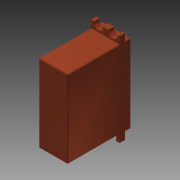
# Autodesk Inventor part: Serwo
Saved by Autodesk Inventor 2014 (Build 180170000, 170)
## iProperties
Created: 2013-10-14
Part Number: Serwo
Material: Miedź
Document SubType Name: Modeling
Designer: Wojciech
Density: 8.94 g/cm^3
Appearance: Miedź - satynowa
Author: Wojciech
Autodesk Inventor part; units mm, degrees
ref_plane "YZ Plane" through (0, 0, 0) normal (1, 0, 0) x (0, 1, 0)
ref_plane "XZ Plane" through (0, 0, 0) normal (0, 1, 0) x (-1, 0, 0)
ref_plane "XY Plane" through (0, 0, 0) normal (0, 0, 1) x (1, 0, 0)
sketch "Szkic1" plane through (0, 0, 0) normal (0, 1, 0) x (-1, 0, 0)
  line L0 (-10, 27) -> (10, 27)
  line L1 (10, 27) -> (10, -27)
  line L2 (10, -27) -> (-10, -27)
  line L3 (-10, -27) -> (-10, 27)
  line L4 (-10, 27) -> (10, -27) construction
  line L5 (10, 27) -> (-10, -27) construction
  point P0 (0, 0)
  dimension "d0" = 20
  dimension "d1" = 54
  constraints: 12 end point, 2 midpoint, 2 parallel, 1 horizontal, 1 perpendicular
  measures "d0" distance of L1.end L2.end
  measures "d1" distance of L0.end L1.end
extrude "Wyciągnięcie proste1" add sketch "Szkic1" along normal blind 36
sketch "Szkic2" plane through (0, 36, 0) normal (0, 1, 0) x (1, 0, 0)
  line L0 (-10, -27) -> (10, -27) projected
  line L1 (10, -27) -> (10, 27) projected
  line L2 (10, 27) -> (-10, 27) projected
  line L3 (-10, 27) -> (-10, -27) projected
  line L4 (-10, -27) -> (-10, -32)
  line L5 (-10, -32) -> (10, -32)
  line L6 (10, -32) -> (10, -27)
  line L7 (10, 27) -> (10, 32)
  line L8 (10, 32) -> (-10, 32)
  line L9 (-10, 32) -> (-10, 27)
  circle A0 centre (-5.0245, -32) radius 3
  circle A1 centre (5.0062, -32) radius 3
  circle A2 centre (-5.0245, 32) radius 3
  circle A3 centre (5.0062, 32) radius 3
  point P0 (0, 0)
  dimension "d4" = 5
  dimension "d5" = 5
  dimension "d8" = 6
  dimension "d9" = 6
  dimension "d10" = 6
  dimension "d11" = 6
  constraints: 12 end point, 4 centre point, 4 point on line, 3 perpendicular, 2 collinear, 1 coincident, 1 parallel
  measures "d4" distance of L0.start L4.end
  measures "d5" distance of L1.end L7.end
  measures "d8" diameter of A0
  measures "d9" diameter of A1
  measures "d10" diameter of A2
  measures "d11" diameter of A3
extrude "Wyciągnięcie proste2" add sketch "Szkic2" along normal blind 4 contours L3 L2 L1 L0 | L0 L6 L5 A1 A0 L4 | L9 L8 A2 A3 L7 L2 | A0 L5 | L5 A1 | L8 A2 | A3 L8 picked at (-4.1905, -30.6328) picked at (5.8402, -30.6328) picked at (-5.5926, 30.2476) picked at (4.4381, 30.2476)
hole "Otwór1" at (5.2587, 40, 31.3846) direction (0, -1, 0) diameter 6 depth 8 tip angle 118
hole "Otwór2" at (-4.8112, 40, 31.2727) direction (0, -1, 0) diameter 6 depth 8 tip angle 118
hole "Otwór3" at (4.5874, 40, -30.3776) direction (0, -1, 0) diameter 6 depth 8 tip angle 118
hole "Otwór4" at (-4.6993, 40, -30.4895) direction (0, -1, 0) diameter 6 depth 8 tip angle 118
sketch "Szkic3" plane through (0, 40, 0) normal (0, 1, 0) x (1, 0, 0)
  line L0 (-10, 27) -> (10, 27)
  line L1 (10, 27) -> (10, -27)
  line L2 (10, -27) -> (-10, -27)
  line L3 (-10, -27) -> (-10, 27)
  line L4 (-10, 27) -> (10, -27) construction
  line L5 (10, 27) -> (-10, -27) construction
  point P0 (0, 0)
  dimension "d48" = 20
  dimension "d49" = 54
  constraints: 12 end point, 2 midpoint, 2 parallel, 1 horizontal, 1 perpendicular
  measures "d48" distance of L1.end L2.end
  measures "d49" distance of L0.end L1.end
extrude "Wyciągnięcie proste3" add sketch "Szkic3" along normal blind 4
sketch "Szkic4" plane through (0, 44, 0) normal (0, 1, 0) x (1, 0, 0)
  line L0 (-8.5229, 17.6007) -> (8.5229, 17.6007)
  line L1 (8.5229, 17.6007) -> (8.5229, 0)
  line L2 (8.5229, 0) -> (-8.5229, 0)
  line L3 (-8.5229, 0) -> (-8.5229, 17.6007)
  line L4 (-8.5229, 17.6007) -> (8.5229, 0) construction
  line L5 (8.5229, 17.6007) -> (-8.5229, 0) construction
  arc A0 (8.5229, 17.6007) -> (-8.5229, 17.6007) centre (0, 17.6007) ccw
  point P0 (0, 0)
  point P1 (0, 8.8003)
  constraints: 12 end point, 2 midpoint, 2 parallel, 2 point on circle, 2 tangent, 1 centre point, 1 horizontal, 1 perpendicular
extrude "Wyciągnięcie proste4" add sketch "Szkic4" along normal blind 1
sketch "Szkic5" plane through (0, 45, 0) normal (0, 1, 0) x (1, 0, 0)
  arc A0 (8.5229, 17.6007) -> (-8.5229, 17.6007) centre (0, 17.6007) ccw projected
  circle A1 centre (0, 17.6007) radius 5
  point P0 (0, 0)
  dimension "d54" = 10
  constraints: 1 centre point, 1 coincident
  measures "d54" diameter of A1
extrude "Wyciągnięcie proste5" add sketch "Szkic5" along normal blind 1
sketch "Szkic6" plane through (0, 46, -17.6007) normal (0, 1, 0) x (1, 0, 0)
  circle A0 centre (0, 0) radius 5 projected
  circle A1 centre (0, 0) radius 4
  point P0 (0, -17.6007)
  dimension "d57" = 8
  constraints: 1 centre point, 1 coincident
  measures "d57" diameter of A1
extrude "Wyciągnięcie proste6" add sketch "Szkic6" along normal blind 1 contours A1
sketch "Szkic7" plane through (0, 47, -17.6007) normal (0, 1, 0) x (1, 0, 0)
  circle A0 centre (0, 0) radius 4 projected
  circle A1 centre (0, 0) radius 2
  point P0 (0, -17.6007)
  dimension "d60" = 4
  constraints: 1 centre point, 1 coincident
  measures "d60" diameter of A1
extrude "Wyciągnięcie proste7" add sketch "Szkic7" along normal blind 4 contours A1
thread "Gwint1" size "M4x0.7" class "6g" standard "ANSI Metric M Profile" full length
chamfer "Faza1" distance 0.5 angle 45 1 edges at (10, 18, -27)
chamfer "Faza2" distance 0.5 angle 45 1 edges at (-10, 18, -27)
chamfer "Faza3" distance 0.5 angle 45 1 edges at (0, 0, -27)
chamfer "Faza4" distance 0.5 angle 45 1 edges at (10, 0, 0.25)
chamfer "Faza5" distance 0.5 angle 45 1 edges at (10, 18.25, 27)
chamfer "Faza6" distance 0.5 angle 45 1 edges at (10, 44, 0)
chamfer "Faza7" distance 0.5 angle 45 1 edges at (-0.25, 44, -27)
chamfer "Faza8" distance 0.5 angle 45 1 edges at (-10, 44, 0.25)
chamfer "Faza9" distance 0.5 angle 45 1 edges at (0, 44, 27)
chamfer "Faza10" distance 0.5 angle 45 1 edges at (-10, 18, 27)
chamfer "Faza11" distance 0.5 angle 45 1 edges at (-10, 0, 0)
chamfer "Faza12" distance 0.5 angle 45 1 edges at (0, 0, 27)
chamfer "Faza13" distance 0.2 angle 45 3 edges at (-8.5229, 45, -8.8003) (0, 45, -26.1235) (8.5229, 45, -8.8003)
chamfer "Faza14" distance 0.2 angle 45 1 edges at (0, 45, 0)
chamfer "Faza15" distance 0.2 angle 45 3 edges at (8.3229, 45, -8.9003) (0, 45, -25.9235) (-8.3229, 45, -8.9003)
chamfer "Faza16" distance 0.2 angle 45 1 edges at (-5, 46, -17.6007)
chamfer "Faza17" distance 0.2 angle 45 1 edges at (-4, 47, -17.6007)
chamfer "Faza18" distance 0.2 angle 45 1 edges at (-2, 51, -17.6007)
chamfer "Faza19" distance 0.2 angle 45 1 edges at (-4.6993, 40, -27.4895)
chamfer "Faza20" distance 0.2 angle 45 1 edges at (4.5874, 40, -27.3776)
chamfer "Faza21" distance 0.2 angle 45 1 edges at (5.2587, 40, 28.3846)
chamfer "Faza22" distance 0.2 angle 45 1 edges at (-4.8112, 40, 28.2727)
chamfer "Faza23" distance 0.2 angle 45 1 edges at (-4.8112, 36, 28.2727)
chamfer "Faza24" distance 0.2 angle 45 1 edges at (5.2587, 36, 28.3846)
chamfer "Faza25" distance 0.2 angle 45 1 edges at (-4.6993, 36, -27.4895)
chamfer "Faza26" distance 0.2 angle 45 1 edges at (4.5874, 36, -27.3776)
chamfer "Faza27" distance 0.2 angle 45 2 edges at (8.6728, 40, -32) (-0.0245, 40, -32)
chamfer "Faza28" distance 0.2 angle 45 2 edges at (-10, 40, -29.5) (-8.7602, 40, -32)
chamfer "Faza29" distance 0.2 angle 45 1 edges at (10, 40, -29.4)
chamfer "Faza30" distance 0.2 angle 45 1 edges at (-10, 40, 29.5)
chamfer "Faza31" distance 0.2 angle 45 1 edges at (-8.8637, 40, 32)
chamfer "Faza32" distance 0.2 angle 45 1 edges at (0.2118, 40, 32)
chamfer "Faza33" distance 0.2 angle 45 1 edges at (9.1995, 40, 32)
chamfer "Faza34" distance 0.2 angle 45 1 edges at (10, 40, 29.4)
chamfer "Faza35" distance 0.2 angle 45 2 edges at (10, 39.9, 27) (10, 41.75, 27)
chamfer "Faza36" distance 0.2 angle 45 2 edges at (10, 41.75, -27) (10, 39.9, -27)
chamfer "Faza37" distance 0.2 angle 45 2 edges at (-10, 41.75, 27) (-10, 39.9, 27)
chamfer "Faza38" distance 0.2 angle 45 2 edges at (-10, 41.75, -27) (-10, 39.9, -27)
